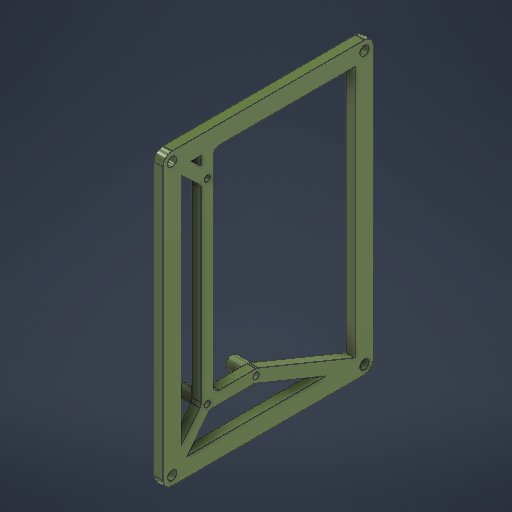
# Autodesk Inventor part: individual_servodriver_support
Saved by Autodesk Inventor 2026.1 (Build 301233000, 233)
## iProperties
Created: 2026-05-02
Part Number: individual_servodriver_support
Material: Generic
Document SubType Name: Modeling
Designer: emanuel
Density: 1 g/cm^3
Appearance: Default
Author: emanuel
Autodesk Inventor part; units mm, degrees
ref_plane "YZ Plane" through (0, 0, 0) normal (1, 0, 0) x (0, 1, 0)
ref_plane "XZ Plane" through (0, 0, 0) normal (0, 1, 0) x (-1, 0, 0)
ref_plane "XY Plane" through (0, 0, 0) normal (0, 0, 1) x (1, 0, 0)
sketch "Sketch1" plane through (0, 0, 0) normal (1, 0, 0) x (0, 1, 0)
  line L0 (0, 0) -> (0, -16)
  circle A0 centre (0, 0) radius 1
  circle A1 centre (0, -16) radius 1
  line L1 (0, 0) -> (64, 0)
  circle A2 centre (64, 0) radius 1
  line L2 (64, 0) -> (0, 0) construction
  line L3 (64, 2) -> (0, 2)
  line L4 (0, -2) -> (64, -2)
  arc A3 (64, -2) -> (64, 2) centre (64, 0) ccw
  arc A4 (0, 2) -> (0, -2) centre (0, 0) ccw
  line L5 (0, 0) -> (0, -16) construction
  line L6 (-2, 0) -> (-2, -16)
  line L7 (2, -16) -> (2, 0)
  arc A5 (2, 0) -> (-2, 0) centre (0, 0) ccw
  arc A6 (-2, -16) -> (2, -16) centre (0, -16) ccw
  point P0 (32, 0)
  point P1 (0, -8)
  point P2 (2, -2)
  dimension "d0" = 16
  dimension "d1" = 2
  dimension "d2" = 2
  dimension "d3" = 64
  dimension "d4" = 2
  dimension "d5" = 4
  dimension "d6" = 4
  constraints: 20 end point, 8 point on circle, 8 tangent, 7 centre point, 4 equal length, 3 coincident, 2 midpoint, 1 horizontal, 1 vertical
  measures "d0" distance of L0.start L0.end
  measures "d1" diameter of A0
  measures "d2" diameter of A1
  measures "d3" distance of L1.start L1.end
  measures "d4" diameter of A2
  measures "d5" diameter of A4
  measures "d6" diameter of A6
extrude "Extrusion1" add sketch "Sketch1" along normal blind 3 contours A0 L1 L7 L4 L0 | L0 A4 A5 L1 A0 | L4 L7 A6 L6 A4 | A5 L3 A3 L4 L7
sketch "Sketch2" plane through (3, 0, 0) normal (1, 0, 0) x (0, 0, -1)
  circle A0 centre (0, 64) radius 1 projected
  circle A1 centre (0, 64) radius 1
  circle A2 centre (0, 64) radius 2
  circle A3 centre (0, 0) radius 1
  circle A4 centre (0, 0) radius 2
  circle A5 centre (16, 0) radius 1 projected
  circle A6 centre (16, 0) radius 1
  circle A7 centre (16, 0) radius 2
  dimension "d9" = 2
  dimension "d10" = 4
  dimension "d11" = 2
  dimension "d12" = 4
  constraints: 6 centre point, 6 coincident
  measures "d9" diameter of A3
  measures "d10" diameter of A4
  measures "d11" diameter of A6
  measures "d12" diameter of A7
extrude "Extrusion2" add sketch "Sketch2" against normal blind 8
sketch "Sketch3" plane through (3, 0, 0) normal (1, 0, 0) x (0, 0, -1)
  arc A0 (0, -2) -> (-2, 0) centre (0, 0) ccw projected
  line L0 (0, 0) -> (0, 30)
  line L1 (0, 30) -> (20, 30)
  line L2 (-11.5, 74.5) -> (51.5, 74.5)
  line L3 (51.5, 74.5) -> (51.5, -14.5)
  line L4 (51.5, -14.5) -> (-11.5, -14.5)
  line L5 (-11.5, -14.5) -> (-11.5, 74.5)
  line L6 (-11.5, 74.5) -> (51.5, -14.5) construction
  line L7 (51.5, 74.5) -> (-11.5, -14.5) construction
  circle A1 centre (-11.5, 74.5) radius 1.5
  circle A2 centre (51.5, 74.5) radius 1.5
  circle A3 centre (51.5, -14.5) radius 1.5
  circle A4 centre (-11.5, -14.5) radius 1.5
  line L8 (-11.5, -14.5) -> (51.5, -14.5) construction
  line L9 (-11.5, -17.5) -> (51.5, -17.5)
  line L10 (51.5, -11.5) -> (-11.5, -11.5)
  arc A5 (-11.5, -11.5) -> (-11.5, -17.5) centre (-11.5, -14.5) ccw
  arc A6 (51.5, -17.5) -> (51.5, -11.5) centre (51.5, -14.5) ccw
  line L11 (51.5, -14.5) -> (51.5, 74.5) construction
  line L12 (54.5, -14.5) -> (54.5, 74.5)
  line L13 (48.5, 74.5) -> (48.5, -14.5)
  arc A7 (48.5, -14.5) -> (54.5, -14.5) centre (51.5, -14.5) ccw
  arc A8 (54.5, 74.5) -> (48.5, 74.5) centre (51.5, 74.5) ccw
  line L14 (51.5, 74.5) -> (-11.5, 74.5) construction
  line L15 (51.5, 77.5) -> (-11.5, 77.5)
  line L16 (-11.5, 71.5) -> (51.5, 71.5)
  arc A9 (51.5, 71.5) -> (51.5, 77.5) centre (51.5, 74.5) ccw
  arc A10 (-11.5, 77.5) -> (-11.5, 71.5) centre (-11.5, 74.5) ccw
  line L17 (-11.5, 74.5) -> (-11.5, -14.5) construction
  line L18 (-14.5, 74.5) -> (-14.5, -14.5)
  line L19 (-8.5, -14.5) -> (-8.5, 74.5)
  arc A11 (-8.5, 74.5) -> (-14.5, 74.5) centre (-11.5, 74.5) ccw
  arc A12 (-14.5, -14.5) -> (-8.5, -14.5) centre (-11.5, -14.5) ccw
  point P0 (20, -14.5)
  point P1 (51.5, 30)
  point P2 (20, 74.5)
  point P3 (-11.5, 30)
  point P4 (-8.5, -11.5)
  point P5 (-8.5, 71.5)
  point P6 (48.5, 71.5)
  point P7 (48.5, -11.5)
  point P8 (54.5, -14.5)
  point P9 (51.5, 77.5)
  point P10 (-14.5, 74.5)
  point P11 (-14.5, -14.5)
  dimension "d15" = 30
  dimension "d16" = 20
  dimension "d17" = 63
  dimension "d18" = 89
  dimension "d19" = 3
  dimension "d20" = 3
  dimension "d21" = 3
  dimension "d22" = 3
  dimension "d23" = 6
  dimension "d24" = 6
  dimension "d25" = 6
  dimension "d26" = 6
  constraints: 48 end point, 16 point on circle, 16 tangent, 12 centre point, 8 equal length, 6 midpoint, 4 coincident, 3 perpendicular, 2 horizontal, 1 vertical
  measures "d15" distance of L0.start L0.end
  measures "d16" distance of L0.end L1.end
  measures "d17" distance of L3.end L4.end
  measures "d18" distance of L2.end L3.end
  measures "d19" diameter of A1
  measures "d20" diameter of A2
  measures "d21" diameter of A3
  measures "d22" diameter of A4
  measures "d23" diameter of A6
  measures "d24" diameter of A8
  measures "d25" diameter of A10
  measures "d26" diameter of A12
extrude "Extrusion3" add sketch "Sketch3" against normal blind 3 contours A1 L5 A10 A11 L2 | L2 L19 L16 L5 A1 | A11 L15 A8 L2 | L2 L13 L16 L19 | L16 L19 L10 L5 | L5 A5 L18 A10 | A8 A9 L3 A2 L2 | L2 A2 L3 L16 L13 | L10 L19 L4 A4 L5 | L5 A4 L4 A12 A5 | L16 L3 L10 L13 | L10 L13 L4 L19 | L10 L3 A3 L4 L13 | A9 L12 A6 L3 | L4 A7 L9 A12 | A6 A7 L4 A3 L3
sketch "Sketch4" plane through (3, 0, 0) normal (1, 0, 0) x (0, 0, -1)
  circle A0 centre (-11.5, 74.5) radius 1.5 projected
  circle A1 centre (0, 64) radius 1 projected
  line L0 (-11.5, 74.5) -> (0, 64) construction
  line L1 (-12.8485, 73.023) -> (-1.3485, 62.523)
  line L2 (1.3485, 65.477) -> (-10.1515, 75.977)
  arc A2 (-10.1515, 75.977) -> (-12.8485, 73.023) centre (-11.5, 74.5) ccw
  arc A3 (-1.3485, 62.523) -> (1.3485, 65.477) centre (0, 64) ccw
  circle A4 centre (0, 0) radius 1 projected
  circle A5 centre (-11.5, -14.5) radius 1.5 projected
  line L3 (0, 0) -> (-11.5, -14.5) construction
  line L4 (-1.567, 1.2428) -> (-13.067, -13.2572)
  line L5 (-9.933, -15.7428) -> (1.567, -1.2428)
  arc A6 (1.567, -1.2428) -> (-1.567, 1.2428) centre (0, 0) ccw
  arc A7 (-13.067, -13.2572) -> (-9.933, -15.7428) centre (-11.5, -14.5) ccw
  circle A8 centre (16, 0) radius 1 projected
  circle A9 centre (51.5, -14.5) radius 1.5 projected
  line L6 (16, 0) -> (51.5, -14.5) construction
  line L7 (15.2437, -1.8515) -> (50.7437, -16.3515)
  line L8 (52.2563, -12.6485) -> (16.7563, 1.8515)
  arc A10 (16.7563, 1.8515) -> (15.2437, -1.8515) centre (16, 0) ccw
  arc A11 (50.7437, -16.3515) -> (52.2563, -12.6485) centre (51.5, -14.5) ccw
  circle A12 centre (51.5, 74.5) radius 1.5 projected
  line L9 (0, 64) -> (51.5, 74.5) construction
  line L10 (0.3995, 62.0403) -> (51.8995, 72.5403)
  line L11 (51.1005, 76.4597) -> (-0.3995, 65.9597)
  arc A13 (-0.3995, 65.9597) -> (0.3995, 62.0403) centre (0, 64) ccw
  arc A14 (51.8995, 72.5403) -> (51.1005, 76.4597) centre (51.5, 74.5) ccw
  line L12 (16, 0) -> (51.5, 74.5) construction
  line L13 (17.8055, -0.8603) -> (53.3055, 73.6397)
  line L14 (49.6945, 75.3603) -> (14.1945, 0.8603)
  arc A15 (14.1945, 0.8603) -> (17.8055, -0.8603) centre (16, 0) ccw
  arc A16 (53.3055, 73.6397) -> (49.6945, 75.3603) centre (51.5, 74.5) ccw
  line L15 (0, 64) -> (0, 74.8995) construction
  line L16 (2, 64) -> (2, 74.8995)
  line L17 (-2, 74.8995) -> (-2, 64)
  arc A17 (-2, 64) -> (2, 64) centre (0, 64) ccw
  arc A18 (2, 74.8995) -> (-2, 74.8995) centre (0, 74.8995) ccw
  point P0 (-5.75, 69.25)
  point P1 (-5.75, -7.25)
  point P2 (33.75, -7.25)
  point P3 (25.75, 69.25)
  point P4 (33.75, 37.25)
  point P5 (-1.3485, 62.523)
  point P6 (0.5973, 66.1629)
  point P7 (47.9689, 71.7389)
  point P8 (18.7162, 1.0509)
  point P9 (-1.3485, 62.523)
  point P10 (0, 69.4498)
  point P11 (-2, 68.5343)
  dimension "d29" = 4
  dimension "d30" = 4
  dimension "d31" = 4
  dimension "d45" = 4
  constraints: 48 end point, 24 point on circle, 24 tangent, 12 centre point, 6 midpoint, 6 parallel, 1 concentric, 1 vertical
  measures "d29" diameter of A11
  measures "d30" diameter of A14
  measures "d31" diameter of A16
  measures "d45" diameter of A18
extrude "Extrusion4" add sketch "Sketch4" against normal blind 3 contours A2 L2 L17 A13 L1 | A13 L11 L2 A3 | L17 L2 L11 A13 | L17 A18 L16 L11 L2 | A3 L2 L11 L16 | L14 A16 A14 L10 | A10 L8 L13 A15 | A15 L13 L8 A11 L7 | A6 L5 A7 L4
fillet "Fillet2" radius 2 6 edges at (1.5, 71.5, -2) (1.5, 63.1178, 2) (1.5, 2, -2) (1.5, -2, -15.6073) (1.5, -2, -0.9664) (1.5, 0.6968, 2)
body "Solid1"
